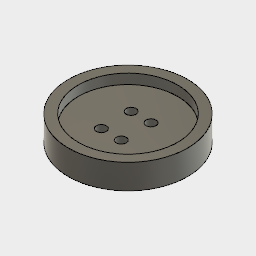
纽扣 (Autodesk Fusion 360 design; units mm, degrees)
Autodesk Fusion 360 part; units mm, degrees
sketch "草图1" plane through (0, 0, 0) normal (0, 1, 0) x (1, 0, 0)
  circle A0 centre (0, 0) radius 10
  circle A1 centre (0, 0) radius 12
  dimension "d1" = 20
  dimension "d2" = 2
  measures "d1" diameter of A0
extrude "拉伸1" add sketch "草图1" along normal blind 3 contours A0 makes body 1
extrude "拉伸2" add sketch "草图1" along normal blind 5 separate body makes body 2
cylinder "圆柱体基本要素1" add diameter 2 height 20 placed x (1, 0, 0) y (0, 0, -1) z (0, 1, 0) at (0, 0, 25) separate body makes body 3
move_body "移动1" bodies 3 to x (1, 0, 0) y (0, 1, 0) z (0, 0, 1) at (0.0076, 0, -25.0072)
pattern_linear "R-阵列1" count 2 spacing 6 along (0, 0, 1) count 2 spacing 4 along (-1, 0, 0) of bodies 3 makes body 4 at (1.0026, 13.3333, 6.0924) makes body 5 at (-2.9974, 13.3333, 0.0924) makes body 6 at (-2.9974, 13.3333, 6.0924)
move_body "移动2" bodies 5 3 4 6 to x (1, 0, 0) y (0, 1, 0) z (0, 0, 1) at (1.7837, 0, -3.11)
move_body "移动3" bodies 3 4 5 6 to x (1, 0, 0) y (0, 1, 0) z (0, 0, 1) at (0.1332, 0, 0.3995)
combine "合并1" operation cut target body 1 tool bodies 3 4 5 6
